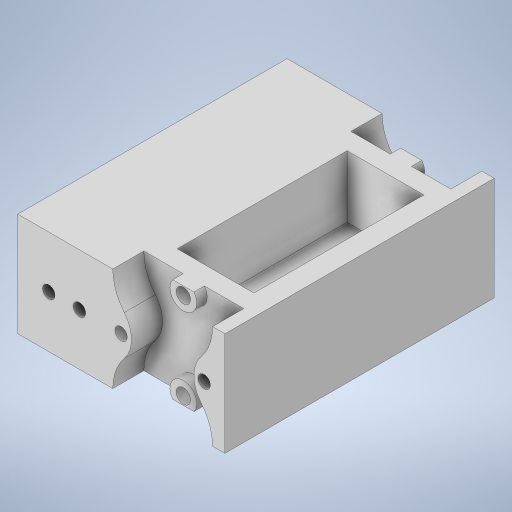
# Autodesk Inventor part: Full_Body
Saved by Autodesk Inventor 2024 (Build 280153000, 153)
## iProperties
Created: 2024-03-19
Part Number: Full_Body
Material: Generic
Document SubType Name: Modeling
Designer: CJ110
Density: 1 g/cm^3
Appearance: Default
Author: CJ110
Autodesk Inventor part; units mm, degrees
ref_plane "YZ Plane" through (0, 0, 0) normal (1, 0, 0) x (0, 1, 0)
sketch "Sketch1" plane through (0, 0, 0) normal (0, 1, 0) x (-1, 0, 0)
  line L0 (0, 0) -> (100, 0)
  line L1 (100, 0) -> (100, 130)
  line L2 (100, 130) -> (0, 130)
  line L3 (0, 130) -> (0, 0)
  dimension "d0" = 130
  dimension "d1" = 100
  constraints: 8 end point, 2 parallel, 1 horizontal, 1 perpendicular
  measures "d0" distance of L0.end L1.end
  measures "d1" distance of L1.end L2.end
extrude "Extrusion1" add sketch "Sketch1" along normal blind 50
sketch "Sketch2" plane through (0, 50, 0) normal (0, 1, 0) x (1, 0, 0)
  line L0 (-47, -106) -> (-10, -106)
  line L1 (-10, -106) -> (-10, -24)
  line L2 (-10, -24) -> (-47, -24)
  line L3 (-47, -24) -> (-47, -106)
  line L4 (0, -130) -> (0, 0) projected
  line L5 (-100, 0) -> (-100, -130) projected
  line L6 (-100, -130) -> (0, -130) projected
  line L7 (0, -130) -> (0, 0) projected
  line L8 (0, 0) -> (-100, 0) projected
  line L9 (-100, -65) -> (0, -65) construction
  point P0 (-47, -65)
  dimension "d4" = 82
  dimension "d5" = 37
  dimension "d6" = 10
  constraints: 10 end point, 3 midpoint, 2 parallel, 1 horizontal, 1 perpendicular, 1 point on line
  measures "d4" distance of L2.end L0.start
  measures "d5" distance of L0.start L0.end
  measures "d6" distance between parallel lines of L4 L1
extrude "Extrusion2" cut sketch "Sketch2" against normal blind 30 contours L3 L2 L1 L0
sketch "Sketch3" plane through (0, 0, 0) normal (0, -1, 0) x (1, 0, 0)
  line L0 (-96, 17.5) -> (-54, 17.5)
  line L1 (-54, 17.5) -> (-54, 112.5)
  line L2 (-54, 112.5) -> (-96, 112.5)
  line L3 (-96, 112.5) -> (-96, 17.5)
  line L4 (-100, 0) -> (-100, 130) projected
  line L5 (0, 0) -> (-100, 0) projected
  line L6 (0, 130) -> (0, 0) projected
  line L7 (-100, 130) -> (0, 130) projected
  line L8 (0, 65) -> (-100, 65) construction
  point P0 (-54, 65)
  dimension "d9" = 42
  dimension "d10" = 95
  dimension "d11" = 4
  constraints: 10 end point, 3 midpoint, 2 horizontal, 2 parallel, 1 perpendicular, 1 point on line
  measures "d9" distance of L0.start L0.end
  measures "d10" distance of L2.end L0.start
  measures "d11" distance between parallel lines of L4 L3
extrude "Extrusion3" cut sketch "Sketch3" against normal blind 27 contours L3 L2 L1 L0
ref_plane "Work Plane1" through (0, 25, 0) normal (0, 1, 0) x (1, 0, 0)
ref_plane "Work Plane2" through (0, 0, 65) normal (0, 0, -1) x (-1, 0, 0)
sketch "Sketch5" plane through (0, 0, 0) normal (0, 0, -1) x (-1, 0, 0)
  line L0 (0, 0) -> (100, 0) projected
  line L1 (100, 0) -> (100, 50) projected
  line L2 (0, 50) -> (100, 50) projected
  line L3 (0, 0) -> (0, 50) projected
  line L4 (-20, 25) -> (120, 25) projected
  arc A0 (0, 10) -> (0, 40) centre (0, 25) ccw
  arc A1 (48.5688, 34.5933) -> (11.5312, 34.5933) centre (30.05, 50) ccw
  arc A2 (11.5312, 15.4067) -> (48.5688, 15.4067) centre (30.05, 0) ccw
  circle A3 centre (60.1, 25) radius 15
  point P0 (54.1397, 50)
  point P1 (5.9603, 50)
  point P2 (5.9603, 0)
  point P3 (54.1397, 0)
  dimension "d14" = 30
  dimension "d15" = 60.1
  constraints: 10 point on circle, 6 point on line, 4 centre point, 3 tangent, 2 equal radius, 2 midpoint
  measures "d14" diameter of A0
  measures "d15" distance of point (0, 25) A3.centre
extrude "Extrusion4" cut sketch "Sketch5" against normal blind 15 contours A2 A0 L4 A3 L0 | A0 A1 L2 A3 L4
mirror "Mirror1" about plane through (0, 0, 65) normal (0, 0, -1) of "Extrusion4"
sketch "Sketch6" plane through (0, 0, 15) normal (0, 0, -1) x (-1, 0, 0)
  arc A0 (48.5688, 34.5933) -> (54.1397, 50) centre (30.05, 50) ccw projected
  line L0 (5.9603, 50) -> (54.1397, 50) projected
  arc A1 (5.9603, 50) -> (11.5312, 34.5933) centre (30.05, 50) ccw projected
  arc A2 (11.5312, 15.4067) -> (11.5312, 34.5933) centre (0, 25) ccw projected
  arc A3 (11.5312, 15.4067) -> (5.9603, 0) centre (30.05, 0) ccw projected
  line L1 (54.1397, 0) -> (5.9603, 0) projected
  arc A4 (54.1397, 0) -> (48.5688, 15.4067) centre (30.05, 0) ccw projected
  arc A5 (48.5688, 34.5933) -> (48.5688, 15.4067) centre (60.1, 25) ccw projected
  arc A6 (24.9265, 50) -> (35.1735, 50) centre (30.05, 46) ccw
  arc A7 (35.1735, 0) -> (24.9265, 0) centre (30.05, 4) ccw
  line L2 (30.05, 50) -> (30.05, 0) construction
  line L3 (-20, 25) -> (120, 25) projected
  circle A8 centre (30.05, 4) radius 3.5
  circle A9 centre (30.05, 46) radius 3.5
  point P0 (0, 0)
  dimension "d18" = 13
  dimension "d19" = 42
  dimension "d20" = 21
  dimension "d21" = 7
  constraints: 6 point on line, 4 centre point, 4 point on circle, 2 coincident, 2 end point, 2 equal radius, 1 vertical
  measures "d18" diameter of A7
  measures "d19" distance of A6.centre A7.centre
  measures "d20" distance from line of L3 A6.centre
  measures "d21" diameter of A8
extrude "Extrusion5" add sketch "Sketch6" along normal blind 5 contours A6 L0 | L1 A7
mirror "Mirror2" about plane through (0, 0, 65) normal (0, 0, -1) of "Extrusion5"
sketch "Sketch7" plane through (-100, 0, 0) normal (0, 0, -1) x (-1, 0, 0)
  circle A0 centre (-90, 25) radius 3
  circle A1 centre (-49.9, 25) radius 3
  arc A2 (-88.4688, 15.4067) -> (-94.0397, 0) centre (-69.95, 0) ccw projected
  arc A3 (-88.4688, 15.4067) -> (-88.4688, 34.5933) centre (-100, 25) ccw projected
  arc A4 (-94.0397, 50) -> (-88.4688, 34.5933) centre (-69.95, 50) ccw projected
  line L0 (-100, 50) -> (-94.0397, 50) projected
  line L1 (-100, 0) -> (-100, 50) projected
  line L2 (-100, 0) -> (-94.0397, 0) projected
  arc A5 (-45.8603, 0) -> (-51.4312, 15.4067) centre (-69.95, 0) ccw projected
  line L3 (-45.8603, 0) -> (0, 0) projected
  line L4 (0, 0) -> (0, 50) projected
  line L5 (-45.8603, 50) -> (0, 50) projected
  arc A6 (-51.4312, 34.5933) -> (-45.8603, 50) centre (-69.95, 50) ccw projected
  arc A7 (-51.4312, 34.5933) -> (-51.4312, 15.4067) centre (-39.9, 25) ccw projected
  line L6 (-120, 25) -> (20, 25) projected
  line L7 (-69.95, 0) -> (-69.95, 50) construction
  circle A8 centre (-29.8, 25) radius 3
  circle A9 centre (-15, 25) radius 3
  dimension "d24" = 6
  dimension "d25" = 6
  dimension "d26" = 40.1
  dimension "d27" = 20.05
  dimension "d30" = 20.1
  dimension "d31" = 14.8
  constraints: 4 centre point, 4 point on line, 2 end point, 2 equal radius, 1 vertical
  measures "d24" diameter of A0
  measures "d25" diameter of A1
  measures "d26" distance of A1.centre A0.centre
  measures "d27" distance from line of L7 A1.centre
  measures "d30" distance of A1.centre A8.centre
  measures "d31" distance of A8.centre A9.centre
extrude "Extrusion6" cut sketch "Sketch7" against normal blind 10 contours L6 A0 | A0 L6 | L6 A1 | A1 L6 | A8 L6 | L6 A8 | A9 L6 | L6 A9
mirror "Mirror3" about plane through (0, 0, 65) normal (0, 0, -1) of "Extrusion6"
equation "\"d20\" = 0.5 * d19"
equation "\"d27\" = 0.5 * d26"
body "Solid1"
